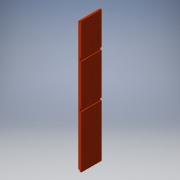
# Autodesk Inventor part: Door Side
Saved by Autodesk Inventor 2016 (Build 200138000, 138)
## iProperties
Created: 2017-10-31
Part Number: Door Side
Material: Wood (Oak)
Document SubType Name: Modeling
Designer: mathaetaes
Density: 0.76 g/cm^3
Appearance: White Oak - Natural Medium Gloss
Author: mathaetaes
Autodesk Inventor part; units mm, degrees
ref_plane "YZ Plane" through (0, 0, 0) normal (1, 0, 0) x (0, 1, 0)
ref_plane "XZ Plane" through (0, 0, 0) normal (0, 1, 0) x (-1, 0, 0)
ref_plane "XY Plane" through (0, 0, 0) normal (0, 0, 1) x (1, 0, 0)
sketch "Sketch1" plane through (0, 0, 0) normal (0, 1, 0) x (-1, 0, 0)
  line L0 (0, 0) -> (-19.05, 0)
  line L1 (-19.05, 0) -> (-19.05, 133.35)
  line L2 (-19.05, 133.35) -> (0, 133.35)
  line L3 (0, 133.35) -> (0, 0)
  dimension "d0" = 19.05
  dimension "d1" = 133.35
  constraints: 8 end point, 2 parallel, 1 horizontal, 1 perpendicular
  measures "d0" distance of L1.end L2.end
  measures "d1" distance of L0.end L1.end
extrude "Board" add sketch "Sketch1" along normal blind 838.2
sketch "Sketch2" plane through (19.05, 0, 133.35) normal (1, 0, 0) x (0, 0, -1)
  line L0 (0, 349.25) -> (133.35, 349.25)
  line L1 (133.35, 349.25) -> (133.35, 330.2)
  line L2 (133.35, 330.2) -> (0, 330.2)
  line L3 (0, 330.2) -> (0, 349.25)
  line L4 (0, 0) -> (133.35, 0) projected
  line L5 (0, 0) -> (0, 838.2) projected
  line L6 (133.35, 0) -> (133.35, 838.2) projected
  line L7 (0, 635) -> (133.35, 635)
  line L8 (133.35, 635) -> (133.35, 615.95)
  line L9 (133.35, 615.95) -> (0, 615.95)
  line L10 (0, 615.95) -> (0, 635)
  line L11 (0, 838.2) -> (133.35, 838.2) projected
  dimension "d4" = 19.05
  dimension "d5" = 330.2
  dimension "d9" = 19.05
  dimension "d13" = 203.2
  dimension "d14" = 266.7
  constraints: 16 end point, 4 collinear, 4 parallel, 2 horizontal, 2 perpendicular
  measures "d4" distance of L0.end L1.end
  measures "d5" distance between parallel lines of L4 L2
  measures "d9" distance of L7.end L8.end
  measures "d13" distance between parallel lines of L7 L11
  measures "d14" distance between parallel lines of L0 L9
extrude "Extrusion2" cut sketch "Sketch2" against normal blind 9.525 contours L0 L1 L2 L3 | L5 L7 L6 L9
sketch "Sketch3" plane through (0, 838.2, 0) normal (0, 1, 0) x (1, 0, 0)
  line L0 (0, -133.35) -> (19.05, -133.35) projected
  line L1 (19.05, -133.35) -> (9.525, -133.35)
  line L2 (9.525, -133.35) -> (9.525, 0)
  line L3 (9.525, 0) -> (19.05, 0)
  line L4 (19.05, 0) -> (19.05, -133.35)
  line L5 (19.05, 0) -> (0, 0) projected
  dimension "d15" = 9.525
  constraints: 8 end point, 2 parallel, 1 collinear, 1 horizontal, 1 perpendicular
  measures "d15" distance of L2.end L3.end
extrude "Extrusion3" add sketch "Sketch3" along normal blind 9.525
sketch "Sketch4" plane through (0, 0, 0) normal (0, -1, 0) x (1, 0, 0)
  line L0 (19.05, 0) -> (9.525, 0)
  line L1 (9.525, 0) -> (9.525, 133.35)
  line L2 (9.525, 133.35) -> (19.05, 133.35)
  line L3 (19.05, 133.35) -> (19.05, 0)
  line L4 (19.05, 0) -> (19.05, 133.35) projected
  line L5 (0, 0) -> (19.05, 0) projected
  line L6 (19.05, 133.35) -> (0, 133.35) projected
  dimension "d18" = 9.525
  constraints: 8 end point, 3 collinear, 2 parallel, 1 horizontal, 1 perpendicular
  measures "d18" distance of L0.start L0.end
extrude "Extrusion4" add sketch "Sketch4" along normal blind 9.525
sketch "Sketch5" plane through (0, 0, 0) normal (-1, 0, 0) x (0, 0, 1)
  line L0 (0, 666.75) -> (11.1125, 666.75)
  line L1 (14.2875, 663.575) -> (14.2875, 631.825)
  line L2 (11.1125, 628.65) -> (0, 628.65)
  line L3 (0, 628.65) -> (0, 666.75)
  line L4 (0, 247.65) -> (11.1125, 247.65)
  line L5 (14.2875, 244.475) -> (14.2875, 212.725)
  line L6 (11.1125, 209.55) -> (0, 209.55)
  line L7 (0, 209.55) -> (0, 247.65)
  line L8 (0, 0) -> (0, 838.2) projected
  line L9 (133.35, 857.25) -> (0, 857.25) projected
  arc A0 (11.1125, 628.65) -> (14.2875, 631.825) centre (11.1125, 631.825) ccw
  arc A1 (14.2875, 663.575) -> (11.1125, 666.75) centre (11.1125, 663.575) ccw
  arc A2 (11.1125, 209.55) -> (14.2875, 212.725) centre (11.1125, 212.725) ccw
  arc A3 (14.2875, 244.475) -> (11.1125, 247.65) centre (11.1125, 244.475) ccw
  point P0 (14.2875, 628.65)
  point P1 (14.2875, 666.75)
  point P2 (14.2875, 209.55)
  point P3 (14.2875, 247.65)
  dimension "d21" = 14.2875
  dimension "d22" = 38.1
  dimension "d23" = 14.2875
  dimension "d24" = 38.1
  dimension "d25" = 190.5
  dimension "d26" = 838.2
  dimension "d27" = 381
  dimension "d28" = 3.175
  constraints: 16 end point, 8 point on circle, 8 point on line, 8 tangent, 4 centre point, 4 parallel, 3 equal radius, 2 collinear, 2 horizontal, 2 perpendicular
  measures "d21" distance of point (14.287, 628.65) L2.end
  measures "d22" distance of point (14.287, 666.75) point (14.287, 628.65)
  measures "d23" distance of point (14.288, 209.55) L6.end
  measures "d24" distance of point (14.288, 247.65) point (14.288, 209.55)
  measures "d25" distance between parallel lines of L0 L9
  measures "d26" distance of L8.start L8.end
  measures "d27" distance between parallel lines of L4 L2
  measures "d28" radius of A0
extrude "Extrusion5" cut sketch "Sketch5" against normal blind 3.175
equation "\"d9\" = d4"
equation "\"d23\" = d21"
equation "\"d24\" = d22"
equation "\"d25\" = 0.25 * d26 - 0.5 * d22"
equation "\"d27\" = 2 * d25"
body "Solid1"
